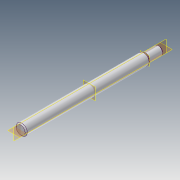
# Autodesk Inventor part: J005526
Saved by Autodesk Inventor 2015 SP1 (Build 190203100, 203)
## iProperties
Created: 2014-11-19
Material: ALUMINUM, 2024-T4/T351
Vendor: HHMI: JFRC - ID&F
Document SubType Name: Modeling
Designer: ARNOLDJ
Density: 2.78 g/cm^3
Description: NRB DRIVE SHAFT
Project: P-242301
Mass: 9.84367 g
Surface Area: 10.745 cm^2
Volume: 1.23046 cm^3
Appearance: Metal-AL-6061 (Machined)
Part Number: J005526
RuleStatus: InUse
AfterDocSave0: file://Part Number Cleaner
LAB/DEPT: DUDMAN (LAB)
REQUESTING SCIENTIST: CODDINGTON, LUKE
SURFACE ROUGHNESS: N/A
DESIGN DEPARTMENT: HHMI: JRC - ID&F
SPECIAL FINISH: NONE
ALTERED ITEM PART NUMBER: 9061K33
ALTERED ITEM VENDOR: MCMASTER CARR
ALTERED ITEM DESCRIPTION: High-Strength 2024 Aluminum Tight Tolerance, 1/4" Diameter, length 1 foot
Revision Number: A
Autodesk Inventor part; units mm, degrees
sketch "Sketch1" plane through (0, 0, 0) normal (0, 0, 1) x (1, 0, 0)
  circle A0 centre (0, 0) radius 3.175
  dimension "d0" = 6.35
  constraints: 1 centre point, 1 coincident
  measures "d0" diameter of A0
extrude "Extrusion1" add sketch "Sketch1" along normal blind 39.3954 and the other way blind 40.2844
ref_plane "Work Plane1" through (0, 0, -31.8262) normal (0, 0, 1) x (1, 0, 0)
sketch "Sketch2" plane through (0, 0, -31.8262) normal (0, 0, 1) x (1, 0, 0)
  circle A0 centre (0, 0) radius 2
  circle A1 centre (0, 0) radius 3.27
  dimension "d9" = 4
  dimension "d10" = 1.27
  constraints: 2 centre point, 2 coincident
  measures "d9" diameter of A0
  measures "d10" radial gap between concentric circles of A1 A0
extrude "Extrusion2" cut sketch "Sketch2" along normal mid plane 1.143
sketch "Sketch3" plane through (0, 0, -40.2844) normal (0, 0, -1) x (-1, 0, 0)
  circle A0 centre (0, 0) radius 3.175 projected
  circle A1 centre (0, 0) radius 3.175
  circle A2 centre (0, 0) radius 2.4892
  dimension "d13" = 4.9784
  dimension "d14" = 0
  constraints: 2 centre point, 2 coincident
  measures "d13" diameter of A2
  measures "d14" radial gap between concentric circles of A0 A1
extrude "Extrusion3" cut sketch "Sketch3" against normal up to next
chamfer "Chamfer1" distance 0.635 angle 45 2 edges at (-3.175, 0, 39.3954) (2.4892, 0, -40.2844)
body "Solid1"
